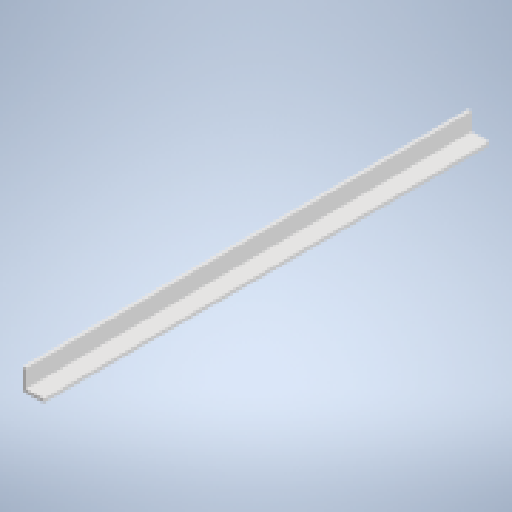
# Autodesk Inventor part: IntakeSlideMiddle
Saved by Autodesk Inventor 2023 (Build 270158000, 158)
## iProperties
Created: 2022-09-16
Part Number: IntakeSlideMiddle
Material: Generic
Document SubType Name: Modeling
Designer: deli
Density: 1 g/cm^3
Appearance: Default
Author: deli
Autodesk Inventor part; units mm, degrees
ref_plane "YZ Plane" through (0, 0, 0) normal (1, 0, 0) x (0, 1, 0)
ref_plane "XZ Plane" through (0, 0, 0) normal (0, 1, 0) x (-1, 0, 0)
ref_plane "XY Plane" through (0, 0, 0) normal (0, 0, 1) x (1, 0, 0)
sketch "Sketch1" plane through (0, 0, 0) normal (0, 0, 1) x (1, 0, 0)
  line L0 (5.5438, 8.6354) -> (5.5438, -10.4146)
  line L1 (5.5438, -10.4146) -> (24.5938, -10.4146)
  line L2 (24.5938, -10.4146) -> (24.5938, -7.2396)
  line L3 (24.5938, -7.2396) -> (8.7188, -7.2396)
  line L4 (8.7188, -7.2396) -> (8.7188, 8.6354)
  line L5 (8.7188, 8.6354) -> (5.5438, 8.6354)
  point P0 (0, 0)
  dimension "d0" = 19.05
  dimension "d1" = 3.175
  constraints: 12 end point, 7 perpendicular, 1 vertical
  measures "d0" distance of L0.end L1.end
  measures "d1" distance of L1.end L2.end
extrude "Extrusion1" add sketch "Sketch1" along normal blind 400
sketch "Sketch2" plane through (8.7188, -7.2396, 0) normal (1, 0, 0) x (0, 0, -1)
  line L0 (0, -3.175) -> (-400, -3.175) projected
  line L1 (-400, -3.175) -> (-400, 0) projected
  line L2 (-400, 0) -> (-400, 15.875) projected
  circle A0 centre (-385, 10.5) radius 1.6
  circle A1 centre (-200, 10.5) radius 1.6
  circle A2 centre (-15, 10.5) radius 1.6
  line L3 (0, -3.175) -> (0, 0) projected
  line L4 (0, 0) -> (-400, 0) projected
  line L5 (-400, -3.175) -> (-400, 0) projected
  line L6 (0, -3.175) -> (-400, -3.175) projected
  point P0 (0, 7.2396)
  dimension "d4" = 3.2
  dimension "d5" = 15
  dimension "d7" = 3.2
  dimension "d8" = 3.2
  dimension "d11" = 185
  dimension "d12" = 185
  dimension "d15" = 10.5
  dimension "d16" = 10.5
  dimension "d17" = 10.5
  constraints: 3 centre point
  measures "d4" diameter of A0
  measures "d5" distance from line of A0.centre L2
  measures "d7" diameter of A1
  measures "d8" diameter of A2
  measures "d11" distance of A2.centre A1.centre
  measures "d12" distance of A0.centre A1.centre
  measures "d15" distance from line of A0.centre L4
  measures "d16" distance from line of A1.centre L4
  measures "d17" distance from line of A2.centre L4
extrude "Extrusion2" cut sketch "Sketch2" against normal blind 10 contours A0 | A1 | A2
equation "\"d12\" = d11"
equation "\"d16\" = d15"
equation "\"d17\" = d15"
body "Solid1"
